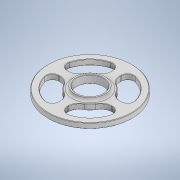
# Autodesk Inventor part: Część21
Saved by Autodesk Inventor 2021 (Build 250183000, 183)
## iProperties
Created: 2023-11-01
Part Number: Część21
Material: Ogólny
Document SubType Name: Modeling
Designer: Jakub
Density: 1 g/cm^3
Appearance: Domyślna
Author: Jakub
Autodesk Inventor part; units mm, degrees
ref_plane "YZ Plane" through (0, 0, 0) normal (1, 0, 0) x (0, 1, 0)
ref_plane "XZ Plane" through (0, 0, 0) normal (0, 1, 0) x (-1, 0, 0)
ref_plane "XY Plane" through (0, 0, 0) normal (0, 0, 1) x (1, 0, 0)
sketch "Szkic1" plane through (0, 0, 0) normal (0, 1, 0) x (-1, 0, 0)
  circle A0 centre (0, 0) radius 15
  circle A1 centre (0, 0) radius 47.5
  dimension "d0" = 30
  dimension "d1" = 95
  constraints: 2 centre point, 2 coincident
  measures "d0" diameter of A0
  measures "d1" diameter of A1
extrude "Wyciągnięcie proste1" add sketch "Szkic1" along normal blind 6
sketch "Szkic2" plane through (0, 6, 0) normal (0, 1, 0) x (1, 0, 0)
  circle A0 centre (0, 0) radius 47.5 projected
  line L0 (0, 47.5) -> (5, 47.5)
  line L1 (5, 47.5) -> (-5, 47.5)
  line L2 (0, -47.5) -> (-5, -47.5)
  line L3 (0, -47.5) -> (5, -47.5) construction
  line L4 (-5, -47.5) -> (5, -47.5)
  line L5 (5, -30.4851) -> (5, -29.1074)
  line L6 (-5, 30.4851) -> (-5, 29.1074)
  line L7 (-47.5, 0) -> (-47.5, 5)
  line L8 (-47.5, 0) -> (-42.5, 0) construction
  line L9 (-47.5, 5) -> (-47.5, -5)
  line L10 (47.5, 0) -> (47.5, 5)
  line L11 (47.5, 0) -> (52.5, 0) construction
  line L12 (47.5, 5) -> (47.5, -5)
  line L13 (-29.1074, -5) -> (-30.4851, -5)
  line L14 (-30.4851, 5) -> (-29.1074, 5)
  line L15 (0, 0) -> (-10.6066, -10.6066)
  circle A1 centre (0, 0) radius 15 projected
  line L16 (0, 0) -> (15, 0) construction
  line L17 (-10.6066, -10.6066) -> (0, 0)
  line L18 (10.6066, 10.6066) -> (0, 0)
  line L19 (10.6066, 10.6066) -> (15.5563, 15.5563)
  line L20 (-10.6066, -10.6066) -> (-15.5563, -15.5563)
  line L21 (0, 0) -> (10.6066, -10.6066)
  line L22 (0, 0) -> (-10.6066, 10.6066)
  line L23 (-10.6066, 10.6066) -> (-15.5563, 15.5563)
  line L24 (10.6066, -10.6066) -> (15.5563, -15.5563)
  line L25 (33.5876, -33.5876) -> (28.6378, -28.6378)
  line L26 (33.5876, 33.5876) -> (28.6378, 28.6378)
  line L27 (-33.5876, 33.5876) -> (-28.6378, 28.6378)
  line L28 (-33.5876, -33.5876) -> (-28.6378, -28.6378)
  arc A2 (28.6378, 28.6378) -> (13.854, 37.2351) centre (5, 5) ccw
  arc A3 (37.2351, 13.854) -> (28.6378, 28.6378) centre (5, 5) ccw
  arc A4 (28.6378, -28.6378) -> (37.2351, -13.854) centre (5, -5) ccw
  arc A5 (13.854, -37.2351) -> (28.6378, -28.6378) centre (5, -5) ccw
  arc A6 (-37.2351, -13.854) -> (-28.6378, -28.6378) centre (-5, -5) ccw
  arc A7 (-28.6378, -28.6378) -> (-13.854, -37.2351) centre (-5, -5) ccw
  arc A8 (-28.6378, 28.6378) -> (-37.2351, 13.854) centre (-5, 5) ccw
  arc A9 (-13.854, 37.2351) -> (-28.6378, 28.6378) centre (-5, 5) ccw
  arc A10 (-11.6526, 18.3647) -> (-15.5563, 15.5563) centre (-5, 5) ccw
  arc A11 (-15.5563, 15.5563) -> (-18.3647, 11.6526) centre (-5, 5) ccw
  arc A12 (-18.3647, -11.6526) -> (-15.5563, -15.5563) centre (-5, -5) ccw
  arc A13 (-15.5563, -15.5563) -> (-11.6526, -18.3647) centre (-5, -5) ccw
  arc A14 (15.5563, -15.5563) -> (18.3647, -11.6526) centre (5, -5) ccw
  arc A15 (11.6526, -18.3647) -> (15.5563, -15.5563) centre (5, -5) ccw
  arc A16 (15.5563, 15.5563) -> (11.6526, 18.3647) centre (5, 5) ccw
  arc A17 (18.3647, 11.6526) -> (15.5563, 15.5563) centre (5, 5) ccw
  arc A18 (-5, 30.4851) -> (-13.854, 37.2351) centre (-12, 30.4851) ccw
  arc A19 (-37.2351, 13.854) -> (-30.4851, 5) centre (-30.4851, 12) ccw
  arc A20 (-30.4851, -5) -> (-37.2351, -13.854) centre (-30.4851, -12) ccw
  arc A21 (-13.854, -37.2351) -> (-5, -30.4851) centre (-12, -30.4851) ccw
  arc A22 (5, -30.4851) -> (13.854, -37.2351) centre (12, -30.4851) ccw
  arc A23 (37.2351, -13.854) -> (30.4851, -5) centre (30.4851, -12) ccw
  arc A24 (30.4851, 5) -> (37.2351, 13.854) centre (30.4851, 12) ccw
  arc A25 (13.854, 37.2351) -> (5, 30.4851) centre (12, 30.4851) ccw
  arc A26 (-11.6526, 18.3647) -> (-5, 29.1074) centre (-17, 29.1074) ccw
  arc A27 (-29.1074, 5) -> (-18.3647, 11.6526) centre (-29.1074, 17) ccw
  arc A28 (-18.3647, -11.6526) -> (-29.1074, -5) centre (-29.1074, -17) ccw
  line L29 (-5, -29.1074) -> (-5, -47.5)
  arc A29 (-5, -29.1074) -> (-11.6526, -18.3647) centre (-17, -29.1074) ccw
  arc A30 (11.6526, -18.3647) -> (5, -29.1074) centre (17, -29.1074) ccw
  line L30 (29.1074, -5) -> (47.5, -5)
  line L31 (5, 47.5) -> (5, 29.1074)
  line L32 (29.1074, 5) -> (47.5, 5)
  arc A31 (5, 29.1074) -> (11.6526, 18.3647) centre (17, 29.1074) ccw
  arc A32 (18.3647, 11.6526) -> (29.1074, 5) centre (29.1074, 17) ccw
  arc A33 (29.1074, -5) -> (18.3647, -11.6526) centre (29.1074, -17) ccw
  point P0 (5, 38.4289)
  point P1 (38.4289, 5)
  point P2 (38.4289, -5)
  point P3 (5, -38.4289)
  point P4 (-38.4289, -5)
  point P5 (-5, -38.4289)
  point P6 (-38.4289, 5)
  point P7 (-5, 38.4289)
  point P8 (-5, 19.9289)
  point P9 (-19.9289, 5)
  point P10 (-19.9289, -5)
  point P11 (-5, -19.9289)
  point P12 (19.9289, -5)
  point P13 (5, -19.9289)
  point P14 (5, 19.9289)
  point P15 (19.9289, 5)
  point P16 (30.4851, -5)
  point P17 (-5, -30.4851)
  dimension "d4" = 5
  dimension "d5" = 10
  dimension "d6" = 5
  dimension "d7" = 180
  dimension "d8" = 10
  dimension "d9" = 5
  dimension "d10" = 90
  dimension "d11" = 10
  dimension "d12" = 5
  dimension "d13" = 90
  dimension "d14" = 10
  dimension "d15" = 135
  dimension "d16" = 7
  dimension "d17" = 7
  dimension "d18" = 7
  dimension "d19" = 7
  dimension "d20" = 7
  dimension "d21" = 7
  dimension "d22" = 7
  dimension "d23" = 12
  dimension "d24" = 12
  dimension "d25" = 12
  constraints: 90 point on circle, 66 end point, 53 point on line, 32 centre point, 32 tangent, 12 coincident, 12 equal radius, 8 horizontal, 4 equal length, 3 vertical, 2 collinear, 1 parallel, 1 perpendicular, 9 other
  measures "d4" distance of L0.start L0.end
  measures "d5" distance of L0.end L1.end
  measures "d6" distance of L2.start L2.end
  measures "d7" angle of L2 L3
  measures "d8" distance of L2.end L4.end
  measures "d9" distance of L7.start L7.end
  measures "d10" angle of L8 L7
  measures "d11" distance of L7.end L9.end
  measures "d12" distance of L10.start L10.end
  measures "d13" angle of L11 L10
  measures "d14" distance of L10.end L12.end
  measures "d15" angle of L15 L16
  measures "d16" distance of L18.start L19.end
  measures "d17" distance of L15.end L20.end
  measures "d18" distance of L22.end L23.end
  measures "d19" distance of L21.end L24.end
  measures "d20" distance of L25.start L25.end
  measures "d21" distance of L26.start L26.end
  measures "d22" radius of A18
  measures "d23" radius of A26
  measures "d24" radius of A29
  measures "d25" radius of A31
extrude "Wyciągnięcie proste2" cut sketch "Szkic2" against normal blind 6 contours A9 A18 L6 A26 A10 A11 A27 L14 A19 A8 | A25 A2 A3 A24 L32 A32 A17 A16 A31 L31 | A6 A20 L13 A28 A12 A13 A29 L29 A21 A7 | A23 A4 A5 A22 L5 A30 A15 A14 A33 L30
sketch "Szkic3" plane through (0, 6, 0) normal (0, 1, 0) x (1, 0, 0)
  circle A0 centre (0, 0) radius 15
  circle A1 centre (0, 0) radius 17
  dimension "d28" = 30
  dimension "d29" = 34
  constraints: 2 centre point, 2 coincident
  measures "d28" diameter of A0
  measures "d29" diameter of A1
extrude "Wyciągnięcie proste3" add sketch "Szkic3" along normal blind 3
fillet "Zaokrąglenie1" radius 3 1 edges at (-17, 6, 0)
chamfer "Faza1" distance 0.5 angle 45 68 edges at (47.5, 6, 0) (47.5, 0, 0) (-36.0518, 6, -7.7561) (-28.6378, 6, -28.6378) (-7.7561, 6, -36.0518) (-5, 6, -29.7962) (-6.7978, 6, -22.7895) (-15.5563, 6, -15.5563) (-22.7895, 6, -6.7978) (-29.7962, 6, -5) (-36.0518, 6, 7.7561) (-29.7962, 6, 5) (-22.7895, 6, 6.7978) (-15.5563, 6, 15.5563) (-6.7978, 6, 22.7895) (-5, 6, 29.7962) (-7.7561, 6, 36.0518) (-28.6378, 6, 28.6378) (7.7561, 6, -36.0518) (28.6378, 6, -28.6378) (36.0518, 6, -7.7561) (29.7962, 6, -5) (22.7895, 6, -6.7978) (15.5563, 6, -15.5563) (6.7978, 6, -22.7895) (5, 6, -29.7962) (15.5563, 6, 15.5563) (22.7895, 6, 6.7978) (29.7962, 6, 5) (36.0518, 6, 7.7561) (28.6378, 6, 28.6378) (7.7561, 6, 36.0518) (5, 6, 29.7962) (6.7978, 6, 22.7895) (7.7561, 0, 36.0518) (28.6378, 0, 28.6378) (36.0518, 0, 7.7561) (29.7962, 0, 5) (22.7895, 0, 6.7978) (15.5563, 0, 15.5563) (6.7978, 0, 22.7895) (5, 0, 29.7962) (-7.7561, 0, 36.0518) (-5, 0, 29.7962) (-6.7978, 0, 22.7895) (-15.5563, 0, 15.5563) (-22.7895, 0, 6.7978) (-29.7962, 0, 5) (-36.0518, 0, 7.7561) (-28.6378, 0, 28.6378) (22.7895, 0, -6.7978) (29.7962, 0, -5) (36.0518, 0, -7.7561) (28.6378, 0, -28.6378) (7.7561, 0, -36.0518) (5, 0, -29.7962) (6.7978, 0, -22.7895) (15.5563, 0, -15.5563) (-28.6378, 0, -28.6378) (-36.0518, 0, -7.7561) (-29.7962, 0, -5) (-22.7895, 0, -6.7978) (-15.5563, 0, -15.5563) (-6.7978, 0, -22.7895) (-5, 0, -29.7962) (-7.7561, 0, -36.0518) (-15, 9, 0) (15, 0, 0)
